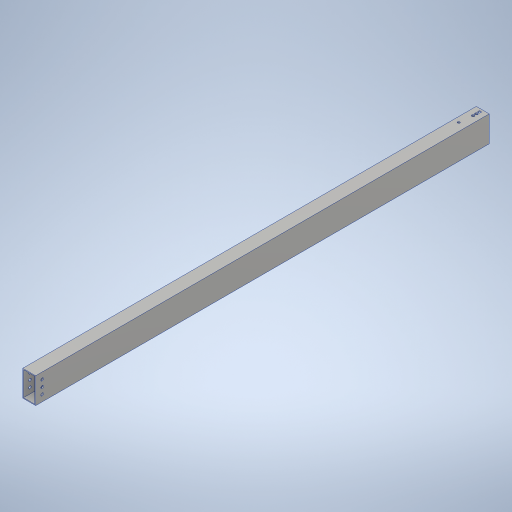
# Autodesk Inventor part: EL2-001
Saved by Autodesk Inventor 2023.4 (Build 274418000, 418)
## iProperties
RuleStatus: InUse
Created: 2025-01-10
Part Number: EL2-001
Material: Aluminum 6061
Document SubType Name: Modeling
Designer: mavericks
Mass: 304.185 g
Surface Area: 718.547 cm^2
Volume: 112.661 cm^3
Density: 2.7 g/cm^3
Appearance: Aluminum - Flat
AfterDocNew0: SHOW
AfterDocOpen0: SHOW
Author: mavericks
Autodesk Inventor part; units mm, degrees
ref_plane "YZ Plane" through (0, 0, 0) normal (1, 0, 0) x (0, 1, 0)
ref_plane "XZ Plane" through (0, 0, 0) normal (0, 1, 0) x (-1, 0, 0)
ref_plane "XY Plane" through (0, 0, 0) normal (0, 0, 1) x (1, 0, 0)
sketch "Sketch1" plane through (0, 0, 0) normal (0, 0, 1) x (1, 0, 0)
  line L0 (-12.7, -25.4) -> (12.7, -25.4)
  line L1 (12.7, -25.4) -> (12.7, 25.4)
  line L2 (12.7, 25.4) -> (-12.7, 25.4)
  line L3 (-12.7, 25.4) -> (-12.7, -25.4)
  line L4 (-12.7, -25.4) -> (12.7, 25.4) construction
  line L5 (12.7, -25.4) -> (-12.7, 25.4) construction
  line L6 (-11.1125, 23.8125) -> (11.1125, 23.8125)
  line L7 (11.1125, 23.8125) -> (11.1125, -23.8125)
  line L8 (11.1125, -23.8125) -> (-11.1125, -23.8125)
  line L9 (-11.1125, -23.8125) -> (-11.1125, 23.8125)
  point P0 (0, 0)
  dimension "width" = 25.4
  dimension "height" = 50.8
  dimension "thickness" = 1.5875
  constraints: 20 end point, 4 parallel, 2 midpoint, 2 perpendicular, 1 horizontal, 3 other
  measures "width" distance of L2.end L1.end
  measures "height" distance of L1.end L0.end
  measures "thickness" distance between parallel lines of L2 L6
extrude "Extrusion1" add sketch "Sketch1" along normal mid plane 889
sketch "Sketch2" plane through (-12.7, 25.4, 444.5) normal (0, 1, 0) x (1, 0, 0)
  line L0 (0, 889) -> (0, 0) projected
  line L1 (0, 889) -> (25.4, 889) projected
  point P0 (12.7, 444.5)
  point P1 (12.7, 882.65)
  point P2 (12.7, 876.3)
  point P3 (12.7, 869.95)
  point P4 (12.7, 889)
  dimension "d5" = 12.7
  dimension "d6" = 6.35
  dimension "d7" = 6.35
  dimension "d8" = 6.35
  constraints: 2 vertical alignment, 1 midpoint
  measures "d5" distance from line of L0 point (12.7, 882.65)
  measures "d6" distance of point (12.7, 889) point (12.7, 882.65)
  measures "d7" distance of point (12.7, 882.65) point (12.7, 876.3)
  measures "d8" distance of point (12.7, 876.3) point (12.7, 869.95)
hole "Hole1" at (0, 25.4, -438.15) at (0, 25.4, -431.8) at (0, 25.4, -425.45) direction (0, -1, 0) diameter 5.1054 end through all clearance for "Flat Head Machine Screw (82)" size "#10" standard "Ansi Unified Screw Threads"
sketch "Sketch3" plane through (-12.7, -25.4, 444.5) normal (-1, 0, 0) x (0, 0, 1)
  line L0 (0, 50.8) -> (0, 0) projected
  point P0 (-444.5, 25.4)
  point P1 (-12.7, 12.7)
  point P2 (-12.7, 25.4)
  point P3 (-12.7, 38.1)
  point P4 (0, 25.4)
  dimension "d16" = 12.7
  dimension "d18" = 12.7
  dimension "d19" = 12.7
  constraints: 2 vertical alignment, 1 horizontal alignment, 1 midpoint
  measures "d16" distance from line of L0 point (-12.7, 12.7)
  measures "d18" distance of point (-12.7, 25.4) point (-12.7, 12.7)
  measures "d19" distance of point (-12.7, 25.4) point (-12.7, 38.1)
hole "Hole2" at (-12.7, -12.7, 431.8) at (-12.7, 0, 431.8) at (-12.7, 12.7, 431.8) direction (1, 0, 0) diameter 5.1054 end through all clearance for "Flat Head Machine Screw (82)" size "#10" standard "Ansi Unified Screw Threads"
sketch "Sketch4" plane through (-12.7, 25.4, 444.5) normal (0, 1, 0) x (1, 0, 0)
  circle A0 centre (9.9314, 844.55) radius 10.3124 construction
  line L0 (0, 889) -> (0, 0) construction
  circle A1 centre (12.7, 869.95) radius 2.5527 construction
  point P0 (12.7, 444.5)
  dimension "d27" = 20.6248
  dimension "d28" = 9.9314
  dimension "d29" = 25.4
  constraints: 1 centre point, 1 coincident
  measures "d27" diameter of A0
  measures "d28" distance from line of A0.centre L0
  measures "d29" vertical distance of A0.centre A1.centre
hole "Hole3" at (-2.7686, 25.4, -400.05) direction (0, -1, 0) diameter 4.445 end through all
sketch "Sketch5" plane through (-12.7, -25.4, 444.5) normal (-1, 0, 0) x (0, 0, 1)
  line L0 (-835.66, 38.1) -> (-863.6, 38.1)
  line L1 (-863.6, 38.1) -> (-863.6, 12.7)
  line L2 (-863.6, 12.7) -> (-835.66, 12.7)
  line L3 (-835.66, 12.7) -> (-835.66, 38.1)
  line L4 (-835.66, 38.1) -> (-863.6, 12.7) construction
  line L5 (-863.6, 38.1) -> (-835.66, 12.7) construction
  line L6 (0, 0) -> (-889, 0) projected
  line L7 (-889, 0) -> (-889, 50.8) projected
  point P0 (-444.5, 25.4)
  point P1 (-849.63, 25.4)
  point P2 (-863.6, 25.4)
  point P3 (-889, 25.4)
  dimension "d37" = 27.94
  dimension "d38" = 25.4
  dimension "d40" = 25.4
  constraints: 12 end point, 4 midpoint, 2 parallel, 1 horizontal, 1 horizontal alignment, 1 perpendicular
  measures "d37" distance of L2.end L1.end
  measures "d38" distance between parallel lines of L0 L2
  measures "d40" distance between parallel lines of L7 L1
extrude "Extrusion2" cut sketch "Sketch5" against normal blind 1.5875
equation "\"d7\" = d6"
equation "\"d8\" = d6"
equation "\"d19\" = d18"
body "Solid1"
